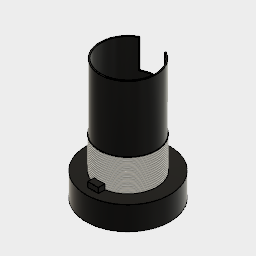
lever1 (Autodesk Fusion 360 design; units mm, degrees)
Autodesk Fusion 360 part; units mm, degrees
sketch "スケッチ6" plane through (0, 0, 0) normal (0, 1, 0) x (1, 0, 0)
  circle A0 centre (0, 0) radius 16
  line L0 (0, -1.75) -> (0, -22.5)
  line L1 (1.75, 0) -> (22.5, 0)
  dimension "d32" = 32
  measures "d32" diameter of A0
extrude "押し出し7" add sketch "スケッチ6" along normal blind 9
sketch "スケッチ7" plane through (0, 0, 0) normal (0, 1, 0) x (1, 0, 0)
  line L0 (0, -1.75) -> (0, -22.5)
  circle A0 centre (0, 0) radius 11
  dimension "d48" = 22
  measures "d48" diameter of A0
extrude "押し出し10" add sketch "スケッチ7" along normal blind 21
ref_plane "作業平面2" through (0, 9, 0) normal (0, 1, 0) x (0, 0, 1)
sketch "スケッチ10" plane through (0, 9, 0) normal (0, 1, 0) x (1, 0, 0)
  line L0 (0, 0, -7.25) -> (0, 0, 13.5)
  line L1 (0, -1.75, -9) -> (0, -22.5, -9)
  line L2 (-2, -10.8) -> (2, -10.8)
  line L3 (2, -10.8) -> (2, -13.3)
  line L4 (2, -13.3) -> (-2, -13.3)
  line L5 (-2, -13.3) -> (-2, -10.8)
  line L6 (0, -1.75) -> (0, -22.5) construction
  dimension "d56" = 10.8
  dimension "d58" = 2.5
  dimension "d59" = 4
  measures "d56" distance of origin L2
  measures "d58" distance of L2.start L4.end
  measures "d59" distance of L3.end L4.end
extrude "押し出し11" add sketch "スケッチ10" along normal blind 2
thread "ねじ3" "ISO Metric profile 22.0 M22x0.75 6g" major diameter 21.908 minor diameter 21.0445 pitch 0.75 angle 60 resizes the face on face at (-3.2009, 13.6667, 10.524)
sketch "スケッチ11" plane through (0, 21, 0) normal (0, 1, 0) x (-1, 0, 0)
  circle A0 centre (0, 0) radius 10.954
  circle A1 centre (0, 0) radius 10.75
  dimension "d62" = 21.5
  measures "d62" diameter of A1
extrude "押し出し12" add sketch "スケッチ11" along normal blind 25 contours A1
sketch "スケッチ12" plane through (0, 46, 0) normal (0, 1, 0) x (-1, 0, 0)
  circle A0 centre (0, 0) radius 10.75
  circle A1 centre (0, 0) radius 10.25
  dimension "d65" = 20.5
  measures "d65" diameter of A1
extrude "押し出し13" cut sketch "スケッチ12" against normal blind 31 contours A1
sketch "スケッチ13" plane through (0, 46, 0) normal (0, 1, 0) x (-1, 0, 0)
  circle A0 centre (0, 0) radius 10.25
  circle A1 centre (0, 0) radius 10.75
  line L0 (0, 1.75, -46) -> (0, 22.5, -46)
  line L1 (0, 0, -44.25) -> (0, 0, -23.5)
  line L2 (-1.75, 0, -46) -> (-22.5, 0, -46)
  line L3 (4.9928, -9) -> (-5.0072, -9)
  line L4 (-5.0072, -9) -> (-5.0072, -16.4603)
  line L5 (-5.0072, -16.4603) -> (4.9928, -16.4603)
  line L6 (4.9928, -16.4603) -> (4.9928, -9)
  dimension "d69" = 10
  dimension "d70" = 9
  measures "d69" distance of L4.end L5.end
  measures "d70" distance of A0.centre L3
extrude "押し出し14" cut sketch "スケッチ13" against normal blind 11 contours A0 A1 L3 L4 L6 | A1 L4 L5 L6 picked at (4.4916, -9.3753)
sketch "スケッチ14" plane through (0, 0, 0) normal (0, -1, 0) x (1, 0, 0)
  circle A0 centre (0, 0) radius 16
  line L0 (-3.8487, 9.5) -> (3.8487, 9.5)
  line L1 (3.8487, 9.5) -> (3.8487, -9.5)
  line L2 (3.8487, -9.5) -> (-3.8487, -9.5)
  line L3 (-3.8487, -9.5) -> (-3.8487, 9.5)
  arc A1 (4.9054, -9) -> (-4.9054, -9) centre (0, 0) ccw
  circle A2 centre (0, 0) radius 10.25
  line L4 (1.75, 0) -> (22.5, 0)
  line L5 (0, 1.75) -> (0, 22.5)
  dimension "d73" = 19
  dimension "d80" = 7.6974
  measures "d73" distance of L0.start L2.end
  measures "d80" distance of L1.end L2.end
extrude "押し出し15" cut sketch "スケッチ14" against normal blind 15 contours L0 L1 L2 L3
sketch "スケッチ15" plane through (0, 0, 0) normal (1, 0, 0) x (0, 0, -1)
  circle A0 centre (0, 4.5) radius 3.5
  line L0 (0, 20, 20) -> (0, 2.5, 20)
  dimension "d77" = 4.5
  dimension "d82" = 7
  measures "d77" distance of origin A0.centre
  measures "d82" diameter of A0
extrude "押し出し16" cut sketch "スケッチ15" along normal mid plane 20
ref_plane "作業平面3" through (1.5, 0, 0) normal (1, 0, 0) x (0, 1, 0)
